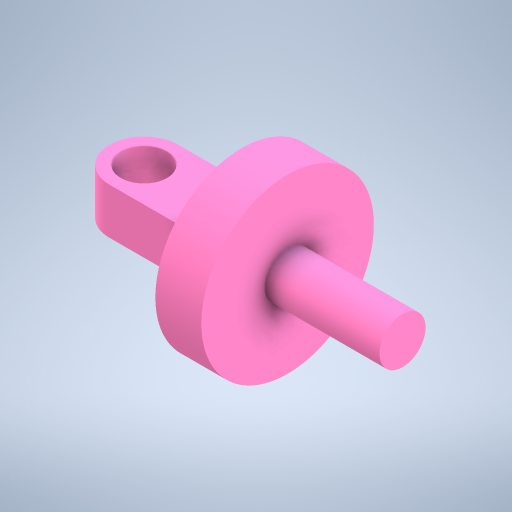
# Autodesk Inventor part: pink-suspension-top
Saved by Autodesk Inventor 2024.1 (Build 281209000, 209)
## iProperties
Created: 2023-11-21
Part Number: pink-suspension-top
Material: ABS プラスチック
Document SubType Name: Modeling
Designer: haruy
Density: 1.06 g/cm^3
Appearance: ピンク
Author: haruy
Autodesk Inventor part; units mm, degrees
ref_plane "YZ Plane" through (0, 0, 0) normal (1, 0, 0) x (0, 1, 0)
ref_plane "XZ Plane" through (0, 0, 0) normal (0, 1, 0) x (-1, 0, 0)
ref_plane "XY Plane" through (0, 0, 0) normal (0, 0, 1) x (1, 0, 0)
sketch "スケッチ1" plane through (0, 0, 0) normal (1, 0, 0) x (0, 1, 0)
  circle A0 centre (0, 0) radius 7.5
  dimension "d0" = 15
  constraints: 1 centre point, 1 coincident
  measures "d0" diameter of A0
extrude "押し出し1" add sketch "スケッチ1" along normal blind 4
sketch "スケッチ2" plane through (0, 0, 0) normal (0, 1, 0) x (-1, 0, 0)
  circle A0 centre (8.5, 0) radius 2
  circle A1 centre (8.5, 0) radius 3
  line L0 (8.5, -3) -> (0, -3)
  line L1 (0, 7.5) -> (0, -7.5) projected
  line L2 (8.5, 3) -> (0, 3)
  point P0 (0, 0)
  dimension "d3" = 4
  dimension "d4" = 6
  dimension "d5" = 8.5
  constraints: 4 end point, 2 centre point, 2 point on circle, 2 point on line, 2 tangent, 1 coincident, 1 horizontal, 1 parallel
  measures "d3" diameter of A0
  measures "d4" diameter of A1
  measures "d5" distance of A0.centre point (0, 0)
extrude "押し出し2" add sketch "スケッチ2" along normal mid plane 4
sketch "スケッチ3" plane through (4, 0, 0) normal (1, 0, 0) x (0, 0, -1)
  circle A0 centre (0, 0) radius 2
  dimension "d8" = 4
  constraints: 1 centre point, 1 coincident
  measures "d8" diameter of A0
extrude "押し出し3" add sketch "スケッチ3" along normal blind 10
